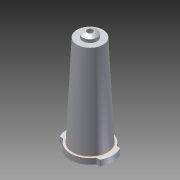
# Autodesk Inventor part: Luer_Female
Saved by Autodesk Inventor 2011 SP2 (Build 150309200, 309)
## iProperties
Created: 2012-02-24
Part Number: Luer_Female
Document SubType Name: Modeling
Designer: sungwook
Density: 1 g/cm^3
Author: sungwook
Autodesk Inventor part; units mm, degrees
ref_plane "YZ Plane" through (0, 0, 0) normal (1, 0, 0) x (0, 1, 0)
ref_plane "XZ Plane" through (0, 0, 0) normal (0, 1, 0) x (-1, 0, 0)
ref_plane "XY Plane" through (0, 0, 0) normal (0, 0, 1) x (1, 0, 0)
sketch "Sketch1" plane through (0, 0, 0) normal (0, 0, 1) x (1, 0, 0)
  circle A0 centre (0, 0) radius 3.365
  dimension "d0" = 6.73
  constraints: 1 centre point, 1 coincident
  measures "d0" diameter of A0
sketch "Sketch2" plane through (0, 0, 0) normal (0, 1, 0) x (-1, 0, 0)
  line L0 (0, -3.16) -> (0, 18.96) projected
  line L1 (0, 0) -> (-2.26, 0)
  line L2 (0, 0) -> (-3, 0)
  line L3 (-3, 0) -> (-2.26, 15.8)
  line L4 (-2.26, 15.8) -> (0, 15.8)
  line L5 (0, 0) -> (0, 15.8)
  dimension "d3" = 2.26
  dimension "d5" = 2.26
  dimension "d6" = 3
  dimension "d7" = 15.8
  constraints: 10 end point, 3 perpendicular, 1 collinear, 1 point on line
  measures "d3" distance of L1.start L1.end
  measures "d5" distance of L4.end L3.end
  measures "d6" distance of L1.start L2.end
  measures "d7" distance of L1.start L4.end
revolve "Revolution1" add sketch "Sketch2" angle 360 about axis through (0, 0, -10) along (0, 0, 1)
sketch "Sketch3" plane through (0, 0, 0) normal (0, 0, -1) x (-1, 0, 0)
  circle A0 centre (0, 0) radius 3 projected
extrude "Extrusion1" add sketch "Sketch1" against normal blind 1
sketch "Sketch4" plane through (0, 0, 0) normal (0, 0, 1) x (1, 0, 0)
  circle A0 centre (0, 0) radius 3.915
  line L0 (0, 1.75) -> (3.5021, 1.75)
  line L1 (8.4729, 1.75) -> (8.4729, -1.75)
  line L2 (3.5021, -1.75) -> (0, -1.75)
  line L3 (0, -1.75) -> (0, 1.75)
  point P0 (0, 0)
  dimension "d11" = 7.83
  dimension "d12" = 3.5
  constraints: 8 end point, 2 coincident, 2 parallel, 2 point on circle, 1 centre point, 1 horizontal, 1 midpoint, 1 perpendicular
  measures "d11" diameter of A0
  measures "d12" distance of L1.end L1.start
extrude "Extrusion2" add sketch "Sketch4" against normal blind 1 contours A0 L2 L3 L0 picked at (1.305, 0)
fillet "Fillet1" radius 0.2 4 edges at (2.8741, 1.75, -0.5) (2.8741, -1.75, -0.5) (3.5021, 1.75, -0.5) (3.5021, -1.75, -0.5)
mirror "Mirror1" about plane through (0, 0, 0) normal (1, 0, 0) of "Extrusion2", "Fillet1"
sketch "Sketch5" plane through (0, 0, -1) normal (0, 0, -1) x (-1, 0, 0)
  arc A0 (-2.817, -1.8406) -> (2.817, -1.8406) centre (0, 0) ccw projected
  circle A1 centre (0, 0) radius 0.205
  dimension "d16" = 0.41
  constraints: 1 centre point, 1 coincident
  measures "d16" diameter of A1
extrude "Extrusion3" [suppressed]
sketch "Sketch6" plane through (0, 0, 0) normal (1, 0, 0) x (0, 1, 0)
  line L0 (0, -10.88) -> (0, 58.28) projected
  line L1 (2.26, 15.8) -> (-2.26, 15.8) projected
  line L2 (0, 16.3531) -> (1.235, 16.3531)
  line L3 (1.235, 16.3531) -> (1.235, 15.8)
  line L4 (1.235, 15.8) -> (0, 15.8)
  line L5 (0, 15.8) -> (0, 16.3531)
  arc A0 (1.235, 16.3531) -> (0, 16.8) centre (0, 14.87) ccw
  line L6 (0, 16.8) -> (0, 16.3531)
  point P0 (0, 0)
  dimension "d19" = 1.235
  constraints: 10 end point, 3 point on line, 2 parallel, 2 point on circle, 1 centre point, 1 collinear, 1 horizontal, 1 perpendicular
  measures "d19" distance between parallel lines of L3 L5
revolve "Revolution2" add sketch "Sketch6" angle 360 about axis through (0, 0, -10) along (0, 0, 1)
sketch "Sketch9" plane through (0, 0, 0) normal (1, 0, 0) x (0, 1, 0)
  line L0 (0, -10.88) -> (0, 58.28) projected
  line L1 (2.26, 15.8) -> (-2.26, 15.8) projected
  line L2 (3, 0) -> (2.26, 15.8) projected
  line L3 (-1.6334, -1) -> (1.6334, -1) projected
  line L4 (0, 18.0112) -> (0, -1)
  line L5 (2.1, -1) -> (1.36, 14.8)
  line L6 (0.5014, 18.0112) -> (0, 18.0112)
  line L7 (0, -1) -> (2.1, -1)
  line L8 (1.36, 14.8) -> (0.5014, 14.8)
  line L9 (0.5014, 14.8) -> (0.5014, 18.0112)
  dimension "d37" = 2.1
  dimension "d38" = 1
  constraints: 12 end point, 4 parallel, 2 point on line, 1 midpoint, 1 perpendicular
  measures "d37" distance of L5.start L4.end
  measures "d38" distance between parallel lines of L1 L8
revolve "Revolution3" cut sketch "Sketch9" angle 360 about axis through (0, 0, -10) along (0, 0, 1)
body "Solid1"
